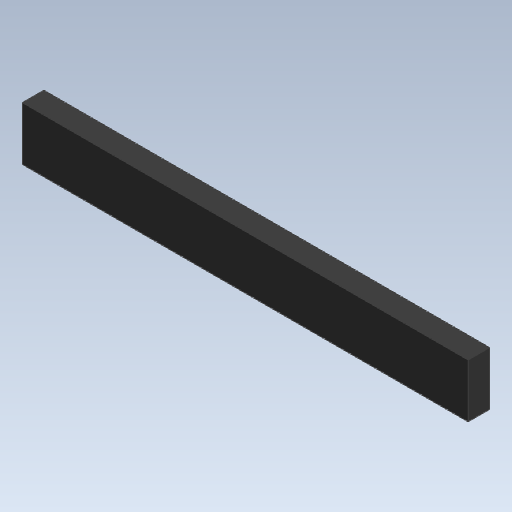
# Autodesk Inventor part: 0 零件
Saved by Autodesk Inventor 2020 (Build 240168000, 168)
## iProperties
Created: 2020-11-03
Part Number: 0 零件
Material: 橡膠
Document SubType Name: Modeling
Designer: p2013
Density: 0.93 g/cm^3
Appearance: 橡膠 - 黑色
Author: p2013
Autodesk Inventor part; units mm, degrees
ref_plane "YZ Plane" through (0, 0, 0) normal (1, 0, 0) x (0, 1, 0)
ref_plane "XZ Plane" through (0, 0, 0) normal (0, 1, 0) x (-1, 0, 0)
ref_plane "XY Plane" through (0, 0, 0) normal (0, 0, 1) x (1, 0, 0)
sketch "草圖1" plane through (0, 0, 0) normal (0, 0, 1) x (1, 0, 0)
  line L0 (0, 0) -> (-46.9602, 0) construction
  line L1 (0, 0) -> (0, 45.4619) construction
  line L2 (-62.5, -7.5) -> (62.5, -7.5)
  line L3 (62.5, -7.5) -> (62.5, 7.5)
  line L4 (62.5, 7.5) -> (-62.5, 7.5)
  line L5 (-62.5, 7.5) -> (-62.5, -7.5)
  line L6 (-62.5, -7.5) -> (62.5, 7.5) construction
  line L7 (62.5, -7.5) -> (-62.5, 7.5) construction
  dimension "d0" = 15
  dimension "d1" = 125
  constraints: 16 end point, 2 horizontal, 2 midpoint, 2 parallel, 1 perpendicular, 1 vertical
  measures "d0" distance between parallel lines of L2 L4
  measures "d1" distance between parallel lines of L3 L5
extrude "擠出1" add sketch "草圖1" along normal mid plane 6
